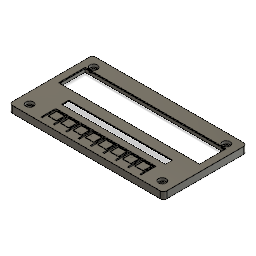
DisplayEnclosure_Front_v1 (Autodesk Fusion 360 design; units mm, degrees)
Autodesk Fusion 360 part; units mm, degrees
sketch "Base" plane through (0, 0, 0) normal (0, 1, 0) x (1, 0, 0)
  line L0 (0, 0) -> (111, 0)
  line L1 (111, 0) -> (111, 60)
  line L2 (111, 60) -> (0, 60)
  line L3 (0, 60) -> (0, 0)
  line L4 (1.6, 1.6) -> (109.4, 1.6) construction
  line L5 (109.4, 1.6) -> (109.4, 58.4) construction
  line L6 (109.4, 58.4) -> (1.6, 58.4) construction
  line L7 (1.6, 58.4) -> (1.6, 1.6) construction
  line L8 (1.6, 58.4) -> (12.6, 58.4) construction
  line L9 (12.6, 58.4) -> (12.6, 47.4) construction
  line L10 (12.6, 47.4) -> (1.6, 47.4) construction
  line L11 (1.6, 47.4) -> (1.6, 58.4) construction
  line L12 (1.6, 1.6) -> (12.6, 1.6) construction
  line L13 (12.6, 1.6) -> (12.6, 12.6) construction
  line L14 (12.6, 12.6) -> (1.6, 12.6) construction
  line L15 (1.6, 12.6) -> (1.6, 1.6) construction
  line L16 (109.4, 1.6) -> (98.4, 1.6) construction
  line L17 (98.4, 1.6) -> (98.4, 12.6) construction
  line L18 (98.4, 12.6) -> (109.4, 12.6) construction
  line L19 (109.4, 12.6) -> (109.4, 1.6) construction
  line L20 (109.4, 58.4) -> (98.4, 58.4) construction
  line L21 (98.4, 58.4) -> (98.4, 47.4) construction
  line L22 (98.4, 47.4) -> (109.4, 47.4) construction
  line L23 (109.4, 47.4) -> (109.4, 58.4) construction
  line L24 (1.6, 58.4) -> (7.9, 58.4) construction
  line L25 (7.9, 58.4) -> (7.9, 53) construction
  line L26 (7.9, 53) -> (1.6, 53) construction
  line L27 (1.6, 53) -> (1.6, 58.4) construction
  line L28 (109.4, 58.4) -> (103.1, 58.4) construction
  line L29 (103.1, 58.4) -> (103.1, 53) construction
  line L30 (103.1, 53) -> (109.4, 53) construction
  line L31 (109.4, 53) -> (109.4, 58.4) construction
  line L32 (109.4, 1.6) -> (103.1, 1.6) construction
  line L33 (103.1, 1.6) -> (103.1, 7) construction
  line L34 (103.1, 7) -> (109.4, 7) construction
  line L35 (109.4, 7) -> (109.4, 1.6) construction
  line L36 (1.6, 1.6) -> (7.9, 1.6) construction
  line L37 (7.9, 1.6) -> (7.9, 7) construction
  line L38 (7.9, 7) -> (1.6, 7) construction
  line L39 (1.6, 7) -> (1.6, 1.6) construction
  circle A0 centre (7.9, 53) radius 1.75
  circle A1 centre (103.1, 53) radius 1.75
  circle A2 centre (103.1, 7) radius 1.75
  circle A3 centre (7.9, 7) radius 1.75
  dimension "d1" = 111
  dimension "d2" = 60
  dimension "d3" = -1.6
  dimension "d4" = 11
  dimension "d5" = 11
  dimension "d6" = 11
  dimension "d7" = 11
  dimension "d8" = 11
  dimension "d9" = 11
  dimension "d10" = 11
  dimension "d11" = 11
  dimension "d12" = 6.3
  dimension "d13" = 5.4
  dimension "d14" = 6.3
  dimension "d15" = 5.4
  dimension "d16" = 6.3
  dimension "d17" = 5.4
  dimension "d18" = 6.3
  dimension "d19" = 5.4
  dimension "d20" = 3.5
  dimension "d21" = 3.5
  dimension "d22" = 3.5
  dimension "d23" = 3.5
  constraint horizontal L0
  constraint vertical L1
  constraint horizontal L2
  constraint vertical L3
  constraint coincident L0.start L3.end
  constraint horizontal L8
  constraint vertical L9
  constraint horizontal L10
  constraint vertical L11
  constraint horizontal L12
  constraint vertical L13
  constraint horizontal L14
  constraint vertical L15
  constraint horizontal L16
  constraint vertical L17
  constraint horizontal L18
  constraint vertical L19
  constraint horizontal L20
  constraint vertical L21
  constraint horizontal L22
  constraint vertical L23
  constraint horizontal L24
  constraint vertical L25
  constraint horizontal L26
  constraint vertical L27
  constraint horizontal L28
  constraint vertical L29
  constraint horizontal L30
  constraint vertical L31
  constraint horizontal L32
  constraint vertical L33
  constraint horizontal L34
  constraint vertical L35
  constraint horizontal L36
  constraint vertical L37
  constraint horizontal L38
  constraint vertical L39
  constraint coincident L25.end L26.start
  constraint coincident L29.end L30.start
  constraint coincident L33.end L34.start
  constraint coincident L37.end L38.start
  measures "d1" distance of L0.start L0.end
  measures "d2" distance of L0.start L2.end
  measures "d4" distance of L6.end L8.end
  measures "d5" distance of L6.end L10.end
  measures "d6" distance of L4.start L12.end
  measures "d7" distance of L4.start L14.end
  measures "d8" distance of L4.end L16.end
  measures "d9" distance of L4.end L18.end
  measures "d10" distance of L5.end L20.end
  measures "d11" distance of L5.end L22.end
  measures "d12" distance of L6.end L24.end
  measures "d13" distance of L6.end L26.end
  measures "d14" distance of L5.end L28.end
  measures "d15" distance of L5.end L30.end
  measures "d16" distance of L4.end L32.end
  measures "d17" distance of L4.end L34.end
  measures "d18" distance of L4.start L36.end
  measures "d19" distance of L4.start L38.end
  measures "d20" diameter of A0
  measures "d21" diameter of A1
  measures "d22" diameter of A2
  measures "d23" diameter of A3
extrude "Extrude1" add sketch "Base" along normal blind 3
sketch "Display" plane through (0, 3, 0) normal (0, 1, 0) x (-1, 0, 0)
  circle A0 centre (-7.9, -7) radius 1.75
  circle A1 centre (-103.1, -53) radius 1.75
  circle A2 centre (-7.9, -53) radius 1.75
  circle A3 centre (-103.1, -7) radius 1.75
  line L0 (0, -60) -> (0, 0)
  line L1 (0, 0) -> (-111, 0)
  line L2 (-111, 0) -> (-111, -60)
  line L3 (-111, -60) -> (0, -60)
  line L4 (-111, -60) -> (-5, -60) construction
  line L5 (-5, -60) -> (-5, -30.8) construction
  line L6 (-5, -30.8) -> (-111, -30.8) construction
  line L7 (-111, -30.8) -> (-111, -60) construction
  line L8 (0, -60) -> (-106, -60) construction
  line L9 (-106, -60) -> (-106, -30.8) construction
  line L10 (-106, -30.8) -> (0, -30.8) construction
  line L11 (0, -30.8) -> (0, -60) construction
  line L12 (-5, -30.8) -> (-106, -30.8)
  line L13 (-106, -30.8) -> (-106, -49.8)
  line L14 (-106, -49.8) -> (-5, -49.8)
  line L15 (-5, -49.8) -> (-5, -30.8)
  line L16 (-111, 0) -> (-19.5, 0) construction
  line L17 (-19.5, 0) -> (-19.5, -23.5) construction
  line L18 (-19.5, -23.5) -> (-111, -23.5) construction
  line L19 (-111, -23.5) -> (-111, 0) construction
  line L20 (0, 0) -> (-93.8, 0) construction
  line L21 (-93.8, 0) -> (-93.8, -23.5) construction
  line L22 (-93.8, -23.5) -> (0, -23.5) construction
  line L23 (0, -23.5) -> (0, 0) construction
  line L24 (-19.5, -23.5) -> (-93.8, -23.5)
  line L25 (-93.8, -23.5) -> (-93.8, -18.5)
  line L26 (-93.8, -18.5) -> (-19.5, -18.5)
  line L27 (-19.5, -18.5) -> (-19.5, -23.5)
  line L28 (-111, 0) -> (-21.8, 0) construction
  line L29 (-21.8, 0) -> (-21.8, -12.4) construction
  line L30 (-21.8, -12.4) -> (-111, -12.4) construction
  line L31 (-111, -12.4) -> (-111, 0) construction
  line L32 (0, 0) -> (-90, 0) construction
  line L33 (-90, 0) -> (-90, -12.4) construction
  line L34 (-90, -12.4) -> (0, -12.4) construction
  line L35 (0, -12.4) -> (0, 0) construction
  line L36 (-21.8, -12.4) -> (-27.8, -12.4) construction
  line L37 (-27.8, -12.4) -> (-27.8, -6.4) construction
  line L38 (-27.8, -6.4) -> (-21.8, -6.4) construction
  line L39 (-21.8, -6.4) -> (-21.8, -12.4) construction
  line L40 (-36.6857, -12.4) -> (-36.6857, -6.4) construction
  line L41 (-30.6857, -12.4) -> (-36.6857, -12.4) construction
  line L42 (-30.6857, -6.4) -> (-30.6857, -12.4) construction
  line L43 (-36.6857, -6.4) -> (-30.6857, -6.4) construction
  line L44 (-45.5714, -12.4) -> (-45.5714, -6.4) construction
  line L45 (-39.5714, -12.4) -> (-45.5714, -12.4) construction
  line L46 (-39.5714, -6.4) -> (-39.5714, -12.4) construction
  line L47 (-45.5714, -6.4) -> (-39.5714, -6.4) construction
  line L48 (-54.4571, -12.4) -> (-54.4571, -6.4) construction
  line L49 (-48.4571, -12.4) -> (-54.4571, -12.4) construction
  line L50 (-48.4571, -6.4) -> (-48.4571, -12.4) construction
  line L51 (-54.4571, -6.4) -> (-48.4571, -6.4) construction
  line L52 (-63.3429, -12.4) -> (-63.3429, -6.4) construction
  line L53 (-57.3429, -12.4) -> (-63.3429, -12.4) construction
  line L54 (-57.3429, -6.4) -> (-57.3429, -12.4) construction
  line L55 (-63.3429, -6.4) -> (-57.3429, -6.4) construction
  line L56 (-72.2286, -12.4) -> (-72.2286, -6.4) construction
  line L57 (-66.2286, -12.4) -> (-72.2286, -12.4) construction
  line L58 (-66.2286, -6.4) -> (-66.2286, -12.4) construction
  line L59 (-72.2286, -6.4) -> (-66.2286, -6.4) construction
  line L60 (-81.1143, -12.4) -> (-81.1143, -6.4) construction
  line L61 (-75.1143, -12.4) -> (-81.1143, -12.4) construction
  line L62 (-75.1143, -6.4) -> (-75.1143, -12.4) construction
  line L63 (-81.1143, -6.4) -> (-75.1143, -6.4) construction
  line L64 (-90, -12.4) -> (-90, -6.4) construction
  line L65 (-84, -12.4) -> (-90, -12.4) construction
  line L66 (-84, -6.4) -> (-84, -12.4) construction
  line L67 (-90, -6.4) -> (-84, -6.4) construction
  line L68 (-21.8, -6.4) -> (-21.8, 0) construction
  line L69 (-21.8, -3.2) -> (-20.8, -3.2) construction
  line L70 (-20.8, -3.2) -> (-20.8, -12.9)
  line L71 (-21.8, -3.2) -> (-90, -3.2) construction
  line L72 (-20.8, -12.9) -> (-28.8, -12.9)
  line L73 (-28.8, -12.9) -> (-28.8, -3.2)
  line L74 (-37.6857, -12.9) -> (-37.6857, -3.2)
  line L75 (-29.6857, -12.9) -> (-37.6857, -12.9)
  line L76 (-29.6857, -3.2) -> (-29.6857, -12.9)
  line L77 (-46.5714, -12.9) -> (-46.5714, -3.2)
  line L78 (-38.5714, -12.9) -> (-46.5714, -12.9)
  line L79 (-38.5714, -3.2) -> (-38.5714, -12.9)
  line L80 (-55.4571, -12.9) -> (-55.4571, -3.2)
  line L81 (-47.4571, -12.9) -> (-55.4571, -12.9)
  line L82 (-47.4571, -3.2) -> (-47.4571, -12.9)
  line L83 (-64.3429, -12.9) -> (-64.3429, -3.2)
  line L84 (-56.3429, -12.9) -> (-64.3429, -12.9)
  line L85 (-56.3429, -3.2) -> (-56.3429, -12.9)
  line L86 (-73.2286, -12.9) -> (-73.2286, -3.2)
  line L87 (-65.2286, -12.9) -> (-73.2286, -12.9)
  line L88 (-65.2286, -3.2) -> (-65.2286, -12.9)
  line L89 (-82.1143, -12.9) -> (-82.1143, -3.2)
  line L90 (-74.1143, -12.9) -> (-82.1143, -12.9)
  line L91 (-74.1143, -3.2) -> (-74.1143, -12.9)
  line L92 (-91, -12.9) -> (-91, -3.2)
  line L93 (-83, -12.9) -> (-91, -12.9)
  line L94 (-83, -3.2) -> (-83, -12.9)
  line L95 (-28.8, -3.2) -> (-29.6857, -3.2)
  line L96 (-37.6857, -3.2) -> (-38.5714, -3.2)
  line L97 (-46.5714, -3.2) -> (-47.4571, -3.2)
  line L98 (-55.4571, -3.2) -> (-56.3429, -3.2)
  line L99 (-64.3429, -3.2) -> (-65.2286, -3.2)
  line L100 (-73.2286, -3.2) -> (-74.1143, -3.2)
  line L101 (-82.1143, -3.2) -> (-83, -3.2)
  line L102 (-91, -3.2) -> (-91.8, -3.2)
  line L103 (-91.8, -3.2) -> (-91.8, -13.7)
  line L104 (-20.8, -3.2) -> (-20, -3.2)
  line L105 (-20, -3.2) -> (-20, -13.7)
  line L106 (-20, -13.7) -> (-91.8, -13.7)
  circle A4 centre (-7.9, -53) radius 2.75
  circle A5 centre (-103.1, -53) radius 2.75
  circle A6 centre (-103.1, -7) radius 2.75
  circle A7 centre (-7.9, -7) radius 2.75
  line L107 (-27.8, -6.4) -> (-21.8, -6.4)
  line L108 (-21.8, -6.4) -> (-21.8, -12.4)
  line L109 (-21.8, -12.4) -> (-27.8, -12.4)
  line L110 (-27.8, -12.4) -> (-27.8, -6.4)
  line L111 (-30.6857, -12.4) -> (-36.6857, -12.4)
  line L112 (-36.6857, -12.4) -> (-36.6857, -6.4)
  line L113 (-36.6857, -6.4) -> (-30.6857, -6.4)
  line L114 (-30.6857, -6.4) -> (-30.6857, -12.4)
  line L115 (-39.5714, -6.4) -> (-45.5714, -6.4)
  line L116 (-45.5714, -6.4) -> (-45.5714, -12.4)
  line L117 (-45.5714, -12.4) -> (-39.5714, -12.4)
  line L118 (-39.5714, -12.4) -> (-39.5714, -6.4)
  line L119 (-48.4571, -12.4) -> (-54.4571, -12.4)
  line L120 (-54.4571, -12.4) -> (-54.4571, -6.4)
  line L121 (-54.4571, -6.4) -> (-48.4571, -6.4)
  line L122 (-48.4571, -6.4) -> (-48.4571, -12.4)
  line L123 (-57.3429, -6.4) -> (-63.3429, -6.4)
  line L124 (-63.3429, -6.4) -> (-63.3429, -12.4)
  line L125 (-63.3429, -12.4) -> (-57.3429, -12.4)
  line L126 (-57.3429, -12.4) -> (-57.3429, -6.4)
  line L127 (-66.2286, -6.4) -> (-72.2286, -6.4)
  line L128 (-72.2286, -6.4) -> (-72.2286, -12.4)
  line L129 (-72.2286, -12.4) -> (-66.2286, -12.4)
  line L130 (-66.2286, -12.4) -> (-66.2286, -6.4)
  line L131 (-75.1143, -12.4) -> (-81.1143, -12.4)
  line L132 (-81.1143, -12.4) -> (-81.1143, -6.4)
  line L133 (-81.1143, -6.4) -> (-75.1143, -6.4)
  line L134 (-75.1143, -6.4) -> (-75.1143, -12.4)
  line L135 (-84, -6.4) -> (-90, -6.4)
  line L136 (-90, -6.4) -> (-90, -12.4)
  line L137 (-90, -12.4) -> (-84, -12.4)
  line L138 (-84, -12.4) -> (-84, -6.4)
  point P0 (-21.8, -3.2)
  dimension "d28" = 106
  dimension "d29" = 29.2
  dimension "d35" = 106
  dimension "d36" = 29.2
  dimension "d37" = 101
  dimension "d38" = 19
  dimension "d39" = 91.5
  dimension "d40" = 23.5
  dimension "d41" = 93.8
  dimension "d42" = 23.5
  dimension "d43" = 5
  dimension "d44" = 89.2
  dimension "d45" = 12.4
  dimension "d46" = 90
  dimension "d47" = 12.4
  dimension "d48" = 6
  dimension "d49" = 6
  dimension "d52" = -62.2
  dimension "d53" = 0
  dimension "d59" = 6.4
  dimension "d60" = 1
  dimension "d61" = 9.7
  dimension "d62" = 8
  dimension "d65" = -62.2
  dimension "d66" = 0
  dimension "d67" = 0.8
  dimension "d68" = 10.5
  dimension "d69" = 0.8
  dimension "d70" = 10.5
  dimension "d81" = 1
  dimension "d82" = 1
  dimension "d83" = 1
  dimension "d84" = 1
  constraint horizontal L4
  constraint vertical L5
  constraint horizontal L6
  constraint vertical L7
  constraint coincident L2.end L3.start
  constraint horizontal L8
  constraint vertical L9
  constraint horizontal L10
  constraint vertical L11
  constraint coincident L0.start L3.end
  constraint horizontal L12
  constraint vertical L13
  constraint horizontal L14
  constraint vertical L15
  constraint horizontal L16
  constraint vertical L17
  constraint horizontal L18
  constraint vertical L19
  constraint coincident L1.end L2.start
  constraint horizontal L20
  constraint vertical L21
  constraint horizontal L22
  constraint vertical L23
  constraint coincident L0.end L1.start
  constraint horizontal L24
  constraint vertical L25
  constraint horizontal L26
  constraint vertical L27
  constraint coincident L21 L25.end
  constraint horizontal L28
  constraint vertical L29
  constraint horizontal L30
  constraint vertical L31
  constraint horizontal L32
  constraint vertical L33
  constraint horizontal L34
  constraint vertical L35
  constraint horizontal L36
  constraint vertical L37
  constraint horizontal L38
  constraint vertical L39
  constraint perpendicular L28 L68
  constraint midpoint P0 L68
  constraint coincident P0 L69.start
  constraint perpendicular L68 L69
  constraint perpendicular L34 L70
  constraint coincident L33 L71.end
  constraint perpendicular L33 L71
  constraint perpendicular L70 L72
  constraint coincident L71 L73.end
  constraint perpendicular L71 L73
  constraint perpendicular L92 L102
  constraint perpendicular L102 L103
  constraint perpendicular L70 L104
  constraint perpendicular L104 L105
  constraint horizontal L107
  constraint vertical L108
  constraint horizontal L109
  constraint vertical L110
  constraint horizontal L111
  constraint vertical L112
  constraint horizontal L113
  constraint vertical L114
  constraint horizontal L115
  constraint vertical L116
  constraint horizontal L117
  constraint vertical L118
  constraint horizontal L119
  constraint vertical L120
  constraint horizontal L121
  constraint vertical L122
  constraint horizontal L123
  constraint vertical L124
  constraint horizontal L125
  constraint vertical L126
  constraint horizontal L127
  constraint vertical L128
  constraint horizontal L129
  constraint vertical L130
  constraint horizontal L131
  constraint vertical L132
  constraint horizontal L133
  constraint vertical L134
  constraint horizontal L135
  constraint vertical L136
  constraint horizontal L137
  constraint vertical L138
  measures "d28" distance of L2.end L4.end
  measures "d29" distance of L2.end L6.end
  measures "d35" distance of L0.start L8.end
  measures "d36" distance of L0.start L10.end
  measures "d37" distance of L5.end L9.end
  measures "d38" distance of L5.end L14.end
  measures "d39" distance of L1.end L16.end
  measures "d40" distance of L1.end L18.end
  measures "d41" distance of L0.end L20.end
  measures "d42" distance of L0.end L22.end
  measures "d43" distance of L17.end L26.end
  measures "d44" distance of L1.end L28.end
  measures "d45" distance of L1.end L30.end
  measures "d46" distance of L0.end L32.end
  measures "d47" distance of L0.end L34.end
  measures "d48" distance of L29.end L36.end
  measures "d49" distance of L29.end L38.end
  measures "d59" distance of L38.end L28.end
  measures "d60" distance of P0 L69.end
  measures "d61" distance of L69.end L70.end
  measures "d62" distance of L70.end L72.end
  measures "d67" distance of L92.end L102.end
  measures "d68" distance of L102.end L103.end
  measures "d69" distance of L69.end L104.end
  measures "d70" distance of L104.end L105.end
extrude "Extrude2" add 1 faces at (40.1589, 0, -22.5864) along direction (0, -1, 0) blind 1.6
sketch "Sketch3" plane through (0, -1.6, 0) normal (0, -1, 0) x (1, 0, 0)
  circle A0 centre (7.9, -7) radius 1.75
  circle A1 centre (103.1, -53) radius 1.75
  circle A2 centre (7.9, -53) radius 1.75
  circle A3 centre (103.1, -7) radius 1.75
  line L0 (0, 0) -> (0, -60)
  line L1 (0, -60) -> (111, -60)
  line L2 (111, -60) -> (111, 0)
  line L3 (111, 0) -> (0, 0)
  line L4 (110.2, -0.8) -> (0.8, -0.8)
  line L5 (0.8, -0.8) -> (0.8, -59.2)
  line L6 (0.8, -59.2) -> (110.2, -59.2)
  line L7 (110.2, -59.2) -> (110.2, -0.8)
  dimension "d56" = -0.8
extrude "Extrude3" cut sketch "Sketch3" against normal blind 3.8 contours L4 L5 L6 L7
extrude "Extrude4" cut sketch "Display" against normal blind 0.8 contours L12 L13 L14 L15 | L24 L25 L26 L27 | L70 L72 L73 L74 L75 L76 L77 L78 L79 L80 L81 L82 L83 L84 L85 L86 L87 L88 L89 L90 L91 L92 L93 L94 L95 L96 L97 L98 L99 L100 L101 L102 L103 L104 L105 L106
sketch "Sketch4" plane through (0, 2.2, 0) normal (0, -1, 0) x (1, 0, 0)
  line L0 (5, -30.8) -> (106, -30.8)
  line L1 (106, -30.8) -> (106, -49.8)
  line L2 (106, -49.8) -> (5, -49.8)
  line L3 (5, -49.8) -> (5, -30.8)
  line L4 (93.8, -18.5) -> (93.8, -23.5)
  line L5 (93.8, -23.5) -> (19.5, -23.5)
  line L6 (19.5, -23.5) -> (19.5, -18.5)
  line L7 (19.5, -18.5) -> (93.8, -18.5)
  line L8 (20.8, -12.9) -> (28.8, -12.9)
  line L9 (28.8, -12.9) -> (28.8, -3.2)
  line L10 (28.8, -3.2) -> (29.6857, -3.2)
  line L11 (29.6857, -3.2) -> (29.6857, -12.9)
  line L12 (29.6857, -12.9) -> (37.6857, -12.9)
  line L13 (37.6857, -12.9) -> (37.6857, -3.2)
  line L14 (37.6857, -3.2) -> (38.5714, -3.2)
  line L15 (38.5714, -3.2) -> (38.5714, -12.9)
  line L16 (38.5714, -12.9) -> (46.5714, -12.9)
  line L17 (46.5714, -12.9) -> (46.5714, -3.2)
  line L18 (46.5714, -3.2) -> (47.4571, -3.2)
  line L19 (47.4571, -3.2) -> (47.4571, -12.9)
  line L20 (47.4571, -12.9) -> (55.4571, -12.9)
  line L21 (55.4571, -12.9) -> (55.4571, -3.2)
  line L22 (55.4571, -3.2) -> (56.3429, -3.2)
  line L23 (56.3429, -3.2) -> (56.3429, -12.9)
  line L24 (56.3429, -12.9) -> (64.3429, -12.9)
  line L25 (64.3429, -12.9) -> (64.3429, -3.2)
  line L26 (64.3429, -3.2) -> (65.2286, -3.2)
  line L27 (65.2286, -3.2) -> (65.2286, -12.9)
  line L28 (65.2286, -12.9) -> (73.2286, -12.9)
  line L29 (73.2286, -12.9) -> (73.2286, -3.2)
  line L30 (73.2286, -3.2) -> (74.1143, -3.2)
  line L31 (74.1143, -3.2) -> (74.1143, -12.9)
  line L32 (74.1143, -12.9) -> (82.1143, -12.9)
  line L33 (82.1143, -12.9) -> (82.1143, -3.2)
  line L34 (82.1143, -3.2) -> (83, -3.2)
  line L35 (83, -3.2) -> (83, -12.9)
  line L36 (83, -12.9) -> (91, -12.9)
  line L37 (91, -12.9) -> (91, -3.2)
  line L38 (91, -3.2) -> (91.8, -3.2)
  line L39 (91.8, -3.2) -> (91.8, -13.7)
  line L40 (91.8, -13.7) -> (20, -13.7)
  line L41 (20, -13.7) -> (20, -3.2)
  line L42 (20, -3.2) -> (20.8, -3.2)
  line L43 (20.8, -3.2) -> (20.8, -12.9)
  circle A0 centre (103.1, -7) radius 1.75
  circle A1 centre (7.9, -53) radius 1.75
  circle A2 centre (7.9, -7) radius 1.75
  circle A3 centre (103.1, -53) radius 1.75
  line L44 (110.2, -59.2) -> (110.2, -0.8)
  line L45 (110.2, -0.8) -> (0.8, -0.8)
  line L46 (0.8, -0.8) -> (0.8, -59.2)
  line L47 (0.8, -59.2) -> (110.2, -59.2)
  line L48 (106, -49.8) -> (106.5, -49.8) construction
  line L49 (106.5, -49.8) -> (106.5, -50.2) construction
  line L50 (106.5, -50.2) -> (106, -50.2) construction
  line L51 (106, -50.2) -> (106, -49.8) construction
  line L52 (19.5, -18.5) -> (4.5, -18.5) construction
  line L53 (4.5, -18.5) -> (4.5, -17.7) construction
  line L54 (4.5, -17.7) -> (19.5, -17.7) construction
  line L55 (19.5, -17.7) -> (19.5, -18.5) construction
  line L56 (106.5, -50.2) -> (4.5, -50.2)
  line L57 (4.5, -50.2) -> (4.5, -17.7)
  line L58 (4.5, -17.7) -> (106.5, -17.7)
  line L59 (106.5, -17.7) -> (106.5, -50.2)
  line L60 (91.8, -13.7) -> (91.8, -0.8)
  line L61 (20, -13.7) -> (20, -0.8)
  line L62 (20, -13.7) -> (91.8, -13.7)
  line L63 (87, -12.9) -> (87, -9.4) construction
  circle A4 centre (87, -9.4) radius 1.75
  circle A5 centre (78.1143, -9.4) radius 1.75
  circle A6 centre (69.2286, -9.4) radius 1.75
  circle A7 centre (60.3429, -9.4) radius 1.75
  circle A8 centre (51.4571, -9.4) radius 1.75
  circle A9 centre (42.5714, -9.4) radius 1.75
  circle A10 centre (33.6857, -9.4) radius 1.75
  circle A11 centre (24.8, -9.4) radius 1.75
  point P0 (87, -12.9)
  dimension "d73" = 0.5
  dimension "d74" = 0.4
  dimension "d75" = 15
  dimension "d76" = 0.8
  dimension "d89" = 3.5
  dimension "d90" = 3.5
  dimension "d93" = -62.2
  dimension "d94" = 0
  constraint horizontal L48
  constraint vertical L49
  constraint horizontal L50
  constraint vertical L51
  constraint coincident L1.end L2.start
  constraint horizontal L52
  constraint vertical L53
  constraint horizontal L54
  constraint vertical L55
  constraint coincident L6.end L7.start
  constraint horizontal L56
  constraint vertical L57
  constraint horizontal L58
  constraint vertical L59
  constraint coincident L39.end L40.start
  constraint coincident L45 L60.end
  constraint perpendicular L45 L60
  constraint coincident L40.end L41.start
  constraint coincident L45 L61.end
  constraint perpendicular L45 L61
  constraint midpoint L36 P0
  constraint coincident P0 L63.start
  constraint perpendicular L36 L63
  constraint coincident L63.end A4.centre
  measures "d73" distance of L1.end L48.end
  measures "d74" distance of L1.end L50.end
  measures "d75" distance of L6.end L52.end
  measures "d76" distance of L6.end L54.end
  measures "d89" distance of P0 L63.end
  measures "d90" diameter of A4
extrude "Extrude6" add sketch "Sketch4" along normal blind 2.8 contours L39 L40 L41 L44 L45 L46 L47 L60 L61 L62
extrude "Extrude7" cut sketch "Display" against normal blind 2 contours A4 | A5 | A6 | A7
extrude "Extrude8" cut sketch "Display" against normal blind 0.2 contours L107 L108 L109 L110 | L111 L112 L113 L114 | L115 L116 L117 L118 | L119 L120 L121 L122 | L123 L124 L125 L126 | L127 L128 L129 L130 | L131 L132 L133 L134 | L135 L136 L137 L138
extrude "Extrude9" add sketch "Sketch4" along normal blind 0.2 contours L8 L9 L10 L11 L12 L13 L14 L15 L16 L17 L18 L19 L20 L21 L22 L23 L24 L25 L26 L27 L28 L29 L30 L31 L32 L33 L34 L35 L36 L37 L38 L42 L43 L45 L60 L61
fillet "Fillet1" radius 2.4 4 edges at (111, 0.7, -60) (111, 0.7, 0) (0, 0.7, 0) (0, 0.7, -60)
fillet "Fillet2" radius 1.6 4 edges at (110.2, -1.1, -59.2) (110.2, -1.1, -0.8) (0.8, -1.1, -59.2) (0.8, -1.1, -0.8)
extrude "Extrude10" add 1 faces at (37.8, -1.6, -59.7333) along direction (0, -1, 0) blind 0.4
